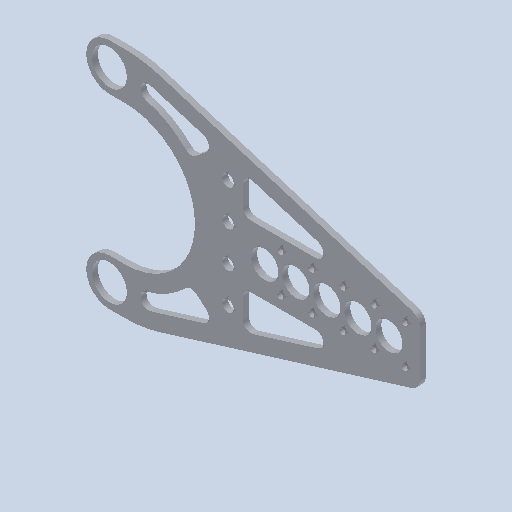
# Autodesk Inventor part: PLATE,END_EFFECTOR,ARM
Saved by Autodesk Inventor 2025.2 (Build 292293000, 293)
## iProperties
ILogicPurgeVersion: 0.0.0.0
OnSaveVersion: 2.2.20.20
Category: _
Manager: _
Created: 2025-03-14
Part Number: PLATE,END_EFFECTOR,ARM
Checked By: 00
Engr Approved By: _
User Status: Work In Process
Material: Polycarbonate, Clear
Description: STANDARD (mm)
Document SubType Name: Sheet Metal
Mfg Approved By: Stephen.Oerton
Designer: John Thibert
Manufacturer: Standard
Standards Organization: Custom
Density: 1.2 g/cm^3
Sheet Metal Rule: Default
Appearance: Polycarbonate - Clear
Mass: 107.961 g
Surface Area: 487.914 cm^2
Volume: 89.9678 cm^3
CN_MASS: 0
CN_SERVICEABLE: _
FIRST_DESCRIPTION: _
SECOND_DESCRIPTION: _
THIRD_DESCRIPTION: _
ModelCat: Uncategorized
Subject: _
Author: John Thibert
Keywords: -
Revision Number: A
Autodesk Inventor part; units mm, degrees
ref_plane "YZ Plane" through (0, 0, 0) normal (1, 0, 0) x (0, 1, 0)
ref_plane "XZ Plane" through (0, 0, 0) normal (0, 1, 0) x (-1, 0, 0)
ref_plane "XY Plane" through (0, 0, 0) normal (0, 0, 1) x (1, 0, 0)
sketch "Sketch2" plane through (0, 0, 0) normal (0, 0, 1) x (1, 0, 0)
  arc A0 (0, -57.15) -> (0, 57.15) centre (0, 0) ccw
  line L0 (241.3, 25.4) -> (241.3, -25.4)
  line L1 (-90.17, 0) -> (296.545, 0) construction
  arc A1 (0, -95.25) -> (28.0159, -91.0367) centre (0, 0) ccw
  arc A2 (28.0159, 91.0367) -> (0, 95.25) centre (0, 0) ccw
  line L2 (28.0159, -91.0367) -> (241.3, -25.4)
  line L3 (241.3, 25.4) -> (28.0159, 91.0367)
  line L4 (0, 95.25) -> (-12.7, 95.25)
  arc A3 (-12.7, 95.25) -> (-12.7, 57.15) centre (-12.7, 76.2) ccw
  line L5 (-12.7, 57.15) -> (0, 57.15)
  line L6 (0, -57.15) -> (-12.7, -57.15)
  arc A4 (-12.7, -57.15) -> (-12.7, -95.25) centre (-12.7, -76.2) ccw
  line L7 (-12.7, -95.25) -> (0, -95.25)
  circle A5 centre (-12.7, -76.2) radius 22.225 construction
  circle A6 centre (-12.7, 76.2) radius 22.225 construction
  dimension "d0" = 114.3
  dimension "d1" = 50.8
  dimension "d4" = 241.3
  dimension "d20" = 12.7
  dimension "d21" = 19.05
  dimension "d63" = 44.45
  measures "d0" diameter of A0
  measures "d1" distance of L0.start L0.end
  measures "d4" distance from line of L0 point (0, 0)
  measures "d20" distance of L4.start L4.end
  measures "d21" radius of A3
  measures "d63" diameter of A5
extrude "Plate1" add sketch "Sketch2" along normal blind 4.7625
sketch "Sketch3" plane through (0, 0, 4.7625) normal (0, 0, 1) x (1, 0, 0)
  line L0 (241.3, 25.4) -> (241.3, -25.4) construction
  line L1 (-86.36, 0) -> (295.91, 0) construction
  line L2 (228.6, 15.875) -> (228.6, -15.875) construction
  point P0 (0, 0)
  point P1 (228.6, 0)
  dimension "d7" = 31.75
  dimension "d8" = 12.7
  constraints: 2 coincident, 2 end point, 1 midpoint, 1 point on line, 1 vertical
  measures "d7" distance of L2.start L2.end
  measures "d8" distance between parallel lines of L0 L2
hole "Hole1" at (228.6, 15.875, 4.7625) at (228.6, -15.875, 4.7625) direction (0, 0, -1) diameter 5.1054 end through all start extended yes clearance for "Flat Head Machine Screw (82)" size "#10" standard "Ansi Unified Screw Threads"
pattern_linear "Rectangular Pattern1" count 5 spacing 25.4 along (-1, 0, 0) of "Hole1"
sketch "Sketch4" plane through (0, 0, 4.7625) normal (0, 0, 1) x (1, 0, 0)
  arc A0 (-12.7, 95.25) -> (-12.7, 57.15) centre (-12.7, 76.2) ccw construction
  arc A1 (-12.7, -57.15) -> (-12.7, -95.25) centre (-12.7, -76.2) ccw construction
  line L0 (-12.7, 76.2) -> (84.2314, 44.45) construction
  line L1 (-86.36, 0) -> (295.91, 0) construction
  line L2 (-12.7, -76.2) -> (84.2314, -44.45) construction
  circle A2 centre (84.2314, 44.45) radius 11.43 construction
  circle A3 centre (-12.7, 76.2) radius 11.43 construction
  line L3 (-9.1421, 87.0621) -> (87.7893, 55.3121) construction
  line L4 (-16.2579, 65.3379) -> (80.6735, 33.5879) construction
  line L5 (84.2314, 14.8167) -> (84.2314, -14.8167) construction
  point P0 (0, 0)
  point P1 (84.2314, 0)
  dimension "d29" = 101.9988
  dimension "d30" = 44.45
  dimension "d38" = 22.86
  dimension "d39" = 29.6333
  dimension "d40" = 29.6333
  dimension "d41" = 29.6333
  constraints: 10 end point, 8 coincident, 4 point on circle, 3 symmetric about line, 3 tangent, 2 centre point, 2 point on line, 1 equal radius, 1 midpoint, 1 parallel, 1 vertical
  measures "d29" distance of L0.start L0.end
  measures "d30" distance from line of L1 L0.end
  measures "d38" diameter of A2
  measures "d39" distance of point (84.231, 44.45) L5.start
  measures "d40" distance of L5.start L5.end
  measures "d41" distance of L2.end point (84.231, -14.817)
hole "Hole2" at (-12.7, 76.2, 4.7625) at (-12.7, -76.2, 4.7625) direction (0, 0, -1) diameter 28.575 end through all start extended yes
hole "Hole3" at (84.2314, 44.45, 4.7625) at (84.2314, -44.45, 4.7625) at (84.2314, 14.8167, 4.7625) at (84.2314, -14.8167, 4.7625) direction (0, 0, -1) diameter 9.525 end through all start extended yes
sketch "Sketch5" plane through (0, 0, 4.7625) normal (0, 0, 1) x (1, 0, 0)
  arc A0 (0, -57.15) -> (0, 57.15) centre (0, 0) ccw construction
  line L0 (-12.7, -57.15) -> (0, -57.15) construction
  arc A1 (-12.7, -57.15) -> (-12.7, -95.25) centre (-12.7, -76.2) ccw construction
  line L1 (0, -95.25) -> (-12.7, -95.25) construction
  arc A2 (0, -95.25) -> (28.0159, -91.0367) centre (0, 0) ccw construction
  line L2 (241.3, -25.4) -> (28.0159, -91.0367) construction
  line L3 (0, 57.15) -> (-12.7, 57.15) construction
  arc A3 (-12.7, 95.25) -> (-12.7, 57.15) centre (-12.7, 76.2) ccw construction
  line L4 (-12.7, 95.25) -> (0, 95.25) construction
  arc A4 (28.0159, 91.0367) -> (0, 95.25) centre (0, 0) ccw construction
  line L5 (28.0159, 91.0367) -> (241.3, 25.4) construction
  line L6 (228.6, 16.0206) -> (96.5218, 56.6667)
  arc A5 (24.2804, 78.8984) -> (12.7, 81.5672) centre (0, 0) ccw
  arc A6 (69.85, 0) -> (53.5082, 44.8987) centre (0, 0) ccw construction
  line L7 (75.3116, 63.194) -> (53.5082, 44.8987)
  line L8 (12.7, 81.5672) -> (12.7, 68.6858)
  line L9 (-86.36, 0) -> (295.91, 0) construction
  line L10 (228.6, 16.0206) -> (228.6, 0)
  line L11 (241.3, 25.4) -> (241.3, -25.4) construction
  arc A7 (53.5082, 44.8987) -> (12.7, 68.6858) centre (0, 0) ccw
  line L12 (75.3116, 63.194) -> (24.2804, 78.8984)
  line L13 (96.5218, 56.6667) -> (96.5218, 25.4)
  line L14 (96.5218, 25.4) -> (198.1218, 25.4)
  line L15 (96.5218, 56.6667) -> (75.3116, 63.194) construction
  dimension "d42" = 12.7
  dimension "d43" = 12.7
  dimension "d44" = 25.4
  dimension "d45" = 50
  dimension "d46" = 12.7
  dimension "d47" = 25.4
  dimension "d48" = 101.6
  constraints: 16 end point, 6 point on circle, 4 point on line, 3 centre point, 2 collinear, 2 perpendicular, 1 parallel, 1 tangent, 1 vertical
  measures "d42" distance between parallel lines of L5 L6
  measures "d43" radial gap between concentric circles of A0 A6
  measures "d44" distance from line of L8 A3.centre
  measures "d45" angle of L7 L8
  measures "d46" distance between parallel lines of L11 L10
  measures "d47" distance between parallel lines of L9 L14
  measures "d48" distance of L13.end L14.end
extrude "Cut1" cut sketch "Sketch5" against normal blind 4.7625
sketch "Sketch6" plane through (0, 0, 4.7625) normal (0, 0, 1) x (1, 0, 0)
  circle A0 centre (228.6, 15.875) radius 2.5527 construction
  circle A1 centre (203.2, -15.875) radius 2.5527 construction
  line L0 (228.6, 15.875) -> (203.2, -15.875) construction
  point P0 (0, 0)
  point P1 (215.9, 0)
  constraints: 2 end point, 1 midpoint
hole "Hole4" at (215.9, 0, 4.7625) direction (0, 0, -1) diameter 22.225 end through all start extended yes
pattern_linear "Rectangular Pattern2" count 5 spacing 25.4 along (-1, 0, 0) of "Hole4"
fillet "Corner Round1" radius 6.35 7 edges at (12.7, 68.6858, 2.3813) (12.7, 81.5672, 2.3813) (53.5082, 44.8987, 2.3813) (75.3116, 63.194, 2.3813) (198.1218, 25.4, 2.3813) (96.5218, 25.4, 2.3813) (96.5218, 56.6667, 2.3813)
mirror "Mirror1" about plane through (0, 0, 0) normal (0, 1, 0) of "Cut1", "Corner Round1"
fillet "Corner Round2" radius 9.525 2 edges at (241.3, 25.4, 2.3813) (241.3, -25.4, 2.3813)
equation "\"d14\" = Thickness"
equation "\"d39\" = d40"
equation "\"d49\" = Thickness"
equation "\"d6\" = Thickness"
equation "\"BendRadius\" = 1.5 * Thickness"
equation "\"BendReliefWidth\" = Thickness"
equation "\"BendReliefDepth\" = 0.5 * Thickness"
equation "\"CornerReliefSize\" = 4 * Thickness"
equation "\"MinimumRemnant\" = 2 * Thickness"
equation "\"TransitionRadius\" = BendRadius"
equation "\"JacobiRadiusSize\" = BendRadius"
equation "\"GapSize\" = Thickness"
equation "\"Thickness\" = 4.7625"
body "Solid1"
